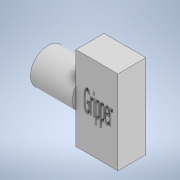
# Autodesk Inventor part: Gripper
Saved by Autodesk Inventor 2020 (Build 240168000, 168)
## iProperties
Created: 2020-12-23
Part Number: Gripper
Material: Generic
Document SubType Name: Modeling
Designer: frost
Density: 1 g/cm^3
Appearance: Default
Author: frost
Autodesk Inventor part; units mm, degrees
ref_plane "YZ Plane" through (0, 0, 0) normal (1, 0, 0) x (0, 1, 0)
ref_plane "XZ Plane" through (0, 0, 0) normal (0, 1, 0) x (-1, 0, 0)
ref_plane "XY Plane" through (0, 0, 0) normal (0, 0, 1) x (1, 0, 0)
sketch "Sketch1" plane through (0, 0, 0) normal (1, 0, 0) x (0, 1, 0)
  circle A0 centre (0, 0) radius 2.5
  dimension "d0" = 5
  constraints: 1 centre point, 1 coincident
  measures "d0" diameter of A0
extrude "Extrusion1" add sketch "Sketch1" along normal blind 6
sketch "Sketch2" plane through (6, 0, 0) normal (1, 0, 0) x (0, 0, -1)
  line L0 (-2, 6) -> (2, 6)
  line L1 (2, 6) -> (2, -6)
  line L2 (2, -6) -> (-2, -6)
  line L3 (-2, -6) -> (-2, 6)
  line L4 (-2, 6) -> (2, -6) construction
  line L5 (2, 6) -> (-2, -6) construction
  point P0 (0, 0)
  dimension "d3" = 4
  dimension "d4" = 12
  constraints: 12 end point, 2 midpoint, 2 parallel, 1 horizontal, 1 perpendicular
  measures "d3" distance of L1.end L2.end
  measures "d4" distance of L0.end L1.end
extrude "Extrusion2" add sketch "Sketch2" along normal blind 6
sketch "Sketch3" plane through (6, 1.5, 2) normal (0, 0, 1) x (1, 0, 0)
  point P0 (-6, -1.5)
sketch "Sketch4" plane through (6, 1.5, 2) normal (0, 0, 1) x (1, 0, 0)
  line L0 (1.137, 0.5676) -> (21.5749, 0.5676) construction
  line L1 (21.5749, 0.5676) -> (21.5749, -3.3796) construction
  line L2 (21.5749, -3.3796) -> (1.137, -3.3796) construction
  line L3 (1.137, -3.3796) -> (1.137, 0.5676) construction
  spline S0 degree 2 poles (1.614, -2.5961) (1.5151, -2.5961) (1.3545, -2.3984) (1.2952, -2.1982) knots 0 0 0 1 2 2 2
  spline S1 degree 2 poles (1.2952, -2.1982) (1.2383, -1.9955) (1.1765, -1.3973) (1.1765, -1.0093) knots 0 0 0 1 2 2 2
  spline S2 degree 2 poles (1.1765, -1.0093) (1.1765, -0.641) (1.2383, -0.0577) (1.2976, 0.1499) knots 0 0 0 1 2 2 2
  spline S3 degree 2 poles (1.2976, 0.1499) (1.352, 0.3501) (1.5176, 0.5676) (1.614, 0.5676) knots 0 0 0 1 2 2 2
  spline S4 degree 2 poles (1.614, 0.5676) (1.661, 0.5676) (1.7475, 0.5231) (1.7845, 0.4836) knots 0 0 0 1 2 2 2
  spline S5 degree 2 poles (1.7845, 0.4836) (1.8167, 0.4539) (1.8933, 0.3452) (1.9155, 0.3056) knots 0 0 0 1 2 2 2
  line L4 (1.9155, 0.3056) -> (1.9155, -0.1838)
  line L5 (1.9155, -0.1838) -> (1.9056, -0.1838)
  spline S6 degree 2 poles (1.9056, -0.1838) (1.8809, -0.117) (1.834, 0.0041) (1.7895, 0.0733) knots 0 0 0 1 2 2 2
  spline S7 degree 2 poles (1.7895, 0.0733) (1.7524, 0.1351) (1.656, 0.2166) (1.5992, 0.2166) knots 0 0 0 1 2 2 2
  spline S8 degree 2 poles (1.5992, 0.2166) (1.4657, 0.2166) (1.3026, -0.4458) (1.3026, -0.9969) knots 0 0 0 1 2 2 2
  spline S9 degree 2 poles (1.3026, -0.9969) (1.3026, -1.3034) (1.3446, -1.7632) (1.3866, -1.9213) knots 0 0 0 1 2 2 2
  spline S10 degree 2 poles (1.3866, -1.9213) (1.4262, -2.0795) (1.5374, -2.2451) (1.6066, -2.2451) knots 0 0 0 1 2 2 2
  spline S11 degree 2 poles (1.6066, -2.2451) (1.6585, -2.2451) (1.7623, -2.1957) (1.7969, -2.1463) knots 0 0 0 1 2 2 2
  line L6 (1.7969, -2.1463) -> (1.7969, -1.3578)
  line L7 (1.7969, -1.3578) -> (1.5843, -1.3578)
  line L8 (1.5843, -1.3578) -> (1.5843, -1.0019)
  line L9 (1.5843, -1.0019) -> (1.918, -1.0019)
  line L10 (1.918, -1.0019) -> (1.918, -2.3341)
  spline S12 degree 2 poles (1.918, -2.3341) (1.8958, -2.3687) (1.8167, -2.475) (1.7821, -2.5071) knots 0 0 0 1 2 2 2
  spline S13 degree 2 poles (1.7821, -2.5071) (1.7376, -2.5516) (1.6659, -2.5961) (1.614, -2.5961) knots 0 0 0 1 2 2 2
  line L11 (2.4247, -0.6608) -> (2.4197, -0.6608)
  spline S14 degree 2 poles (2.4197, -0.6608) (2.4049, -0.6484) (2.3777, -0.6435) (2.358, -0.6435) knots 0 0 0 1 2 2 2
  spline S15 degree 2 poles (2.358, -0.6435) (2.311, -0.6435) (2.2195, -0.7794) (2.1775, -0.9129) knots 0 0 0 1 2 2 2
  line L12 (2.1775, -0.9129) -> (2.1775, -2.5368)
  line L13 (2.1775, -2.5368) -> (2.0614, -2.5368)
  line L14 (2.0614, -2.5368) -> (2.0614, -0.248)
  line L15 (2.0614, -0.248) -> (2.1775, -0.248)
  line L16 (2.1775, -0.248) -> (2.1775, -0.5891)
  spline S16 degree 2 poles (2.1775, -0.5891) (2.2418, -0.4013) (2.3332, -0.248) (2.3777, -0.248) knots 0 0 0 1 2 2 2
  spline S17 degree 2 poles (2.3777, -0.248) (2.395, -0.248) (2.4148, -0.253) (2.4247, -0.2604) knots 0 0 0 1 2 2 2
  line L17 (2.4247, -0.2604) -> (2.4247, -0.6608)
  line L18 (2.6323, -2.5368) -> (2.5161, -2.5368)
  line L19 (2.5161, -2.5368) -> (2.5161, -0.248)
  line L20 (2.5161, -0.248) -> (2.6323, -0.248)
  line L21 (2.6323, -0.248) -> (2.6323, -2.5368)
  line L22 (2.6397, 0.1326) -> (2.5087, 0.1326)
  line L23 (2.5087, 0.1326) -> (2.5087, 0.533)
  line L24 (2.5087, 0.533) -> (2.6397, 0.533)
  line L25 (2.6397, 0.533) -> (2.6397, 0.1326)
  spline S18 degree 2 poles (3.3763, -1.3306) (3.3763, -1.904) (3.2131, -2.5813) (3.0871, -2.5813) knots 0 0 0 1 2 2 2
  spline S19 degree 2 poles (3.0871, -2.5813) (3.0352, -2.5813) (2.9586, -2.5022) (2.9165, -2.4206) knots 0 0 0 1 2 2 2
  line L26 (2.9165, -2.4206) -> (2.9165, -3.3796)
  line L27 (2.9165, -3.3796) -> (2.8004, -3.3796)
  line L28 (2.8004, -3.3796) -> (2.8004, -0.248)
  line L29 (2.8004, -0.248) -> (2.9165, -0.248)
  line L30 (2.9165, -0.248) -> (2.9165, -0.4878)
  spline S20 degree 2 poles (2.9165, -0.4878) (2.9586, -0.3568) (3.0648, -0.1838) (3.1266, -0.1838) knots 0 0 0 1 2 2 2
  spline S21 degree 2 poles (3.1266, -0.1838) (3.2453, -0.1838) (3.3763, -0.8066) (3.3763, -1.3306) knots 0 0 0 1 2 2 2
  spline S22 degree 2 poles (3.2576, -1.3751) (3.2576, -0.9821) (3.1835, -0.5496) (3.0995, -0.5496) knots 0 0 0 1 2 2 2
  spline S23 degree 2 poles (3.0995, -0.5496) (3.05, -0.5496) (2.9586, -0.6954) (2.9165, -0.8091) knots 0 0 0 1 2 2 2
  line L31 (2.9165, -0.8091) -> (2.9165, -2.1092)
  spline S24 degree 2 poles (2.9165, -2.1092) (2.961, -2.1809) (3.0278, -2.2352) (3.0673, -2.2352) knots 0 0 0 1 2 2 2
  spline S25 degree 2 poles (3.0673, -2.2352) (3.1588, -2.2352) (3.2576, -1.7953) (3.2576, -1.3751) knots 0 0 0 1 2 2 2
  spline S26 degree 2 poles (4.0708, -1.3306) (4.0708, -1.904) (3.9077, -2.5813) (3.7816, -2.5813) knots 0 0 0 1 2 2 2
  spline S27 degree 2 poles (3.7816, -2.5813) (3.7297, -2.5813) (3.6531, -2.5022) (3.6111, -2.4206) knots 0 0 0 1 2 2 2
  line L32 (3.6111, -2.4206) -> (3.6111, -3.3796)
  line L33 (3.6111, -3.3796) -> (3.4949, -3.3796)
  line L34 (3.4949, -3.3796) -> (3.4949, -0.248)
  line L35 (3.4949, -0.248) -> (3.6111, -0.248)
  line L36 (3.6111, -0.248) -> (3.6111, -0.4878)
  spline S28 degree 2 poles (3.6111, -0.4878) (3.6531, -0.3568) (3.7594, -0.1838) (3.8212, -0.1838) knots 0 0 0 1 2 2 2
  spline S29 degree 2 poles (3.8212, -0.1838) (3.9398, -0.1838) (4.0708, -0.8066) (4.0708, -1.3306) knots 0 0 0 1 2 2 2
  spline S30 degree 2 poles (3.9522, -1.3751) (3.9522, -0.9821) (3.878, -0.5496) (3.794, -0.5496) knots 0 0 0 1 2 2 2
  spline S31 degree 2 poles (3.794, -0.5496) (3.7445, -0.5496) (3.6531, -0.6954) (3.6111, -0.8091) knots 0 0 0 1 2 2 2
  line L37 (3.6111, -0.8091) -> (3.6111, -2.1092)
  spline S32 degree 2 poles (3.6111, -2.1092) (3.6556, -2.1809) (3.7223, -2.2352) (3.7618, -2.2352) knots 0 0 0 1 2 2 2
  spline S33 degree 2 poles (3.7618, -2.2352) (3.8533, -2.2352) (3.9522, -1.7953) (3.9522, -1.3751) knots 0 0 0 1 2 2 2
  spline S34 degree 2 poles (4.486, -2.5887) (4.3204, -2.5887) (4.14, -1.9732) (4.14, -1.4048) knots 0 0 0 1 2 2 2
  spline S35 degree 2 poles (4.14, -1.4048) (4.14, -0.8462) (4.3155, -0.1838) (4.4589, -0.1838) knots 0 0 0 1 2 2 2
  spline S36 degree 2 poles (4.4589, -0.1838) (4.5206, -0.1838) (4.6195, -0.3074) (4.6566, -0.4384) knots 0 0 0 1 2 2 2
  spline S37 degree 2 poles (4.6566, -0.4384) (4.6937, -0.5694) (4.7332, -0.9475) (4.7332, -1.2219) knots 0 0 0 1 2 2 2
  line L38 (4.7332, -1.2219) -> (4.7332, -1.432)
  line L39 (4.7332, -1.432) -> (4.2562, -1.432)
  spline S38 degree 2 poles (4.2562, -1.432) (4.2562, -1.8299) (4.3773, -2.2525) (4.4836, -2.2525) knots 0 0 0 1 2 2 2
  spline S39 degree 2 poles (4.4836, -2.2525) (4.5231, -2.2525) (4.5948, -2.1957) (4.6245, -2.1512) knots 0 0 0 1 2 2 2
  spline S40 degree 2 poles (4.6245, -2.1512) (4.6566, -2.1018) (4.7011, -2.0153) (4.7134, -1.9757) knots 0 0 0 1 2 2 2
  line L40 (4.7134, -1.9757) -> (4.7208, -1.9757)
  line L41 (4.7208, -1.9757) -> (4.7208, -2.3959)
  spline S41 degree 2 poles (4.7208, -2.3959) (4.7011, -2.4231) (4.6393, -2.5022) (4.617, -2.5244) knots 0 0 0 1 2 2 2
  spline S42 degree 2 poles (4.617, -2.5244) (4.5824, -2.5565) (4.5281, -2.5887) (4.486, -2.5887) knots 0 0 0 1 2 2 2
  spline S43 degree 2 poles (4.617, -1.1378) (4.617, -0.9821) (4.5973, -0.7547) (4.5775, -0.6781) knots 0 0 0 1 2 2 2
  spline S44 degree 2 poles (4.5775, -0.6781) (4.5577, -0.5916) (4.4959, -0.5001) (4.449, -0.5001) knots 0 0 0 1 2 2 2
  spline S45 degree 2 poles (4.449, -0.5001) (4.402, -0.5001) (4.3377, -0.5916) (4.313, -0.6806) knots 0 0 0 1 2 2 2
  spline S46 degree 2 poles (4.313, -0.6806) (4.2858, -0.772) (4.2586, -0.992) (4.2562, -1.1378) knots 0 0 0 1 2 2 2
  line L42 (4.2562, -1.1378) -> (4.617, -1.1378)
  line L43 (5.2152, -0.6608) -> (5.2102, -0.6608)
  spline S47 degree 2 poles (5.2102, -0.6608) (5.1954, -0.6484) (5.1682, -0.6435) (5.1484, -0.6435) knots 0 0 0 1 2 2 2
  spline S48 degree 2 poles (5.1484, -0.6435) (5.1015, -0.6435) (5.01, -0.7794) (4.968, -0.9129) knots 0 0 0 1 2 2 2
  line L44 (4.968, -0.9129) -> (4.968, -2.5368)
  line L45 (4.968, -2.5368) -> (4.8518, -2.5368)
  line L46 (4.8518, -2.5368) -> (4.8518, -0.248)
  line L47 (4.8518, -0.248) -> (4.968, -0.248)
  line L48 (4.968, -0.248) -> (4.968, -0.5891)
  spline S49 degree 2 poles (4.968, -0.5891) (5.0323, -0.4013) (5.1237, -0.248) (5.1682, -0.248) knots 0 0 0 1 2 2 2
  spline S50 degree 2 poles (5.1682, -0.248) (5.1855, -0.248) (5.2053, -0.253) (5.2152, -0.2604) knots 0 0 0 1 2 2 2
  line L49 (5.2152, -0.2604) -> (5.2152, -0.6608)
  point P0 (-6, -1.5)
  constraints: 2 other
extrude "Extrusion3" cut sketch "Sketch4" against normal blind 3
body "Solid1"
